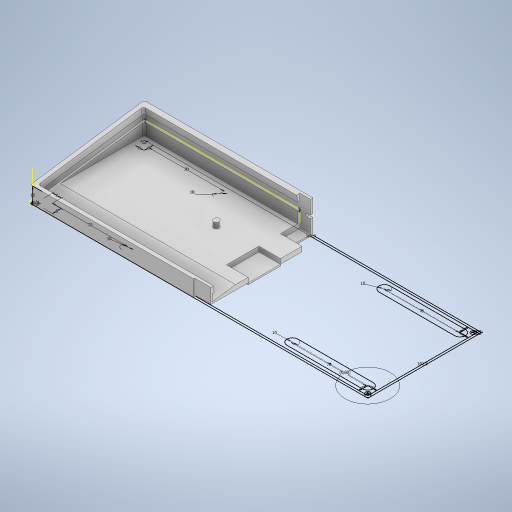
# Autodesk Inventor part: case_in_one_p1
Saved by Autodesk Inventor 2024 (Build 280153000, 153)
## iProperties
Created: 2023-08-03
Part Number: case_in_one_p1
Material: Generic
Document SubType Name: Modeling
Designer: Mika
Density: 1 g/cm^3
Appearance: Default
Author: Mika
Autodesk Inventor part; units mm, degrees
ref_plane "YZ Plane" through (0, 0, 0) normal (1, 0, 0) x (0, 1, 0)
ref_plane "XZ Plane" through (0, 0, 0) normal (0, 1, 0) x (-1, 0, 0)
ref_plane "XY Plane" through (0, 0, 0) normal (0, 0, 1) x (1, 0, 0)
sketch "Sketch1" plane through (0, 0, 0) normal (0, 1, 0) x (-1, 0, 0)
  line L0 (0, 0) -> (-2, 0)
  line L1 (-2, 0) -> (-2, -2)
  line L2 (-2, -2) -> (0, -2)
  line L3 (0, -2) -> (0, 0)
  line L4 (-2, -2) -> (-310.9, -2)
  line L5 (-310.9, -2) -> (-310.9, -103.5)
  line L6 (-308.9, -103.5) -> (-2, -103.5)
  line L7 (-2, -103.5) -> (-2, -2)
  line L8 (-310.9, -103.5) -> (-312.9, -103.5)
  line L9 (-312.9, -103.5) -> (-312.9, -105.5)
  line L10 (-312.9, -105.5) -> (-310.9, -105.5)
  line L11 (-310.9, -105.5) -> (-310.9, -103.5)
  line L12 (-312.9, -105.5) -> (0, -105.5)
  line L13 (0, -105.5) -> (0, 0)
  line L14 (0, 0) -> (-312.9, 0)
  line L15 (-312.9, 0) -> (-312.9, -105.5)
  line L16 (-2, -2) -> (-4, -2)
  line L17 (-4, -2) -> (-4, -4)
  line L18 (-4, -4) -> (-2, -4)
  line L19 (-2, -4) -> (-2, -2)
  line L20 (-2, -103.5) -> (-4, -103.5)
  line L21 (-4, -103.5) -> (-4, -101.5)
  line L22 (-4, -101.5) -> (-2, -101.5)
  line L23 (-2, -101.5) -> (-2, -103.5)
  line L24 (-310.9, -103.5) -> (-308.9, -103.5)
  line L25 (-308.9, -103.5) -> (-308.9, -101.5)
  line L26 (-308.9, -101.5) -> (-310.9, -101.5)
  line L27 (-310.9, -101.5) -> (-310.9, -103.5)
  line L28 (-310.9, -2) -> (-308.9, -2)
  line L29 (-308.9, -2) -> (-308.9, -4)
  line L30 (-308.9, -4) -> (-310.9, -4)
  line L31 (-310.9, -4) -> (-310.9, -2)
  circle A0 centre (-4, -101.5) radius 2
  circle A1 centre (-4, -4) radius 2
  circle A2 centre (-308.9, -4) radius 2
  circle A3 centre (-308.9, -101.5) radius 2
  circle A4 centre (-310.9, -103.5) radius 2
  circle A5 centre (-2, -103.5) radius 2
  circle A6 centre (-2, -2) radius 2
  circle A7 centre (-310.9, -2) radius 2
  line L32 (-2, -2) -> (-10, -2)
  line L33 (-10, -2) -> (-10, -10)
  line L34 (-10, -10) -> (-2, -10)
  line L35 (-2, -10) -> (-2, -2)
  line L36 (-310.9, -2) -> (-302.9, -2)
  line L37 (-302.9, -2) -> (-302.9, -10)
  line L38 (-302.9, -10) -> (-310.9, -10)
  line L39 (-310.9, -10) -> (-310.9, -2)
  line L40 (-310.9, -103.5) -> (-302.9, -103.5)
  line L41 (-302.9, -103.5) -> (-302.9, -95.5)
  line L42 (-302.9, -95.5) -> (-310.9, -95.5)
  line L43 (-310.9, -95.5) -> (-310.9, -103.5)
  line L44 (-2, -103.5) -> (-10, -103.5)
  line L45 (-10, -103.5) -> (-10, -95.5)
  line L46 (-10, -95.5) -> (-2, -95.5)
  line L47 (-2, -95.5) -> (-2, -103.5)
  line L48 (-10, -95.5) -> (-80, -95.5) construction
  line L49 (-10, -90.5) -> (-80, -90.5)
  line L50 (-80, -100.5) -> (-10, -100.5)
  arc A8 (-10, -100.5) -> (-10, -90.5) centre (-10, -95.5) ccw
  arc A9 (-80, -90.5) -> (-80, -100.5) centre (-80, -95.5) ccw
  line L51 (-302.9, -95.5) -> (-232.9, -95.5) construction
  line L52 (-302.9, -100.5) -> (-232.9, -100.5)
  line L53 (-232.9, -90.5) -> (-302.9, -90.5)
  arc A10 (-302.9, -90.5) -> (-302.9, -100.5) centre (-302.9, -95.5) ccw
  arc A11 (-232.9, -100.5) -> (-232.9, -90.5) centre (-232.9, -95.5) ccw
  line L54 (-302.9, -10) -> (-232.9, -10) construction
  line L55 (-302.9, -15) -> (-232.9, -15)
  line L56 (-232.9, -5) -> (-302.9, -5)
  arc A12 (-302.9, -5) -> (-302.9, -15) centre (-302.9, -10) ccw
  arc A13 (-232.9, -15) -> (-232.9, -5) centre (-232.9, -10) ccw
  line L57 (-302.9, -10) -> (-232.9, -10) construction
  line L58 (-10, -10) -> (-80, -10) construction
  line L59 (-10, -5) -> (-80, -5)
  line L60 (-80, -15) -> (-10, -15)
  arc A14 (-10, -15) -> (-10, -5) centre (-10, -10) ccw
  arc A15 (-80, -5) -> (-80, -15) centre (-80, -10) ccw
  point P0 (-2, -105.5)
  point P1 (0, -103.5)
  point P2 (-310.9, 0)
  point P3 (-312.9, -2)
  point P4 (-45, -95.5)
  point P5 (-267.9, -95.5)
  point P6 (-267.9, -10)
  point P7 (-45, -10)
  dimension "d0" = 2
  dimension "d1" = 2
  dimension "d2" = 308.9
  dimension "d3" = 101.5
  dimension "d4" = 2
  dimension "d5" = 2
  dimension "d6" = 2
  dimension "d7" = 2
  dimension "d8" = 2
  dimension "d9" = 2
  dimension "d10" = 2
  dimension "d11" = 2
  dimension "d12" = 2
  dimension "d13" = 2
  dimension "d66" = 8
  dimension "d67" = 8
  dimension "d68" = 8
  dimension "d69" = 8
  dimension "d70" = 8
  dimension "d71" = 8
  dimension "d72" = 8
  dimension "d73" = 8
  dimension "d74" = 70
  dimension "d75" = 10
  dimension "d76" = 70
  dimension "d77" = 10
  dimension "d78" = 70
  dimension "d79" = 0
  dimension "d80" = 10
  dimension "d81" = 70
  dimension "d82" = 10
  constraints: 130 end point, 29 parallel, 18 tangent, 16 point on circle, 14 horizontal, 12 perpendicular, 10 centre point, 8 coincident, 4 midpoint, 2 point on line, 1 collinear, 18 other
  measures "d0" distance of L2.end L1.end
  measures "d1" distance of L1.end L0.end
  measures "d2" distance of L6.end L5.end
  measures "d3" distance of L5.end L4.end
  measures "d4" distance of L10.end L9.end
  measures "d5" distance of L9.end L8.end
  measures "d6" distance of L18.end L17.end
  measures "d7" distance of L17.end L16.end
  measures "d8" distance of L21.end L22.end
  measures "d9" distance of L20.end L21.end
  measures "d10" distance of L26.end L25.end
  measures "d11" distance of L6.start L25.end
  measures "d12" distance of L29.end L30.end
  measures "d13" distance of L28.end L29.end
  measures "d66" distance of L34.end L33.end
  measures "d67" distance of L33.end L32.end
  measures "d68" distance of L37.end L38.end
  measures "d69" distance of L36.end L37.end
  measures "d70" distance of L42.end L41.end
  measures "d71" distance of L41.end L40.end
  measures "d72" distance of L45.end L46.end
  measures "d73" distance of L44.end L45.end
  measures "d74" distance of L45.end L48.end
  measures "d75" diameter of A9
  measures "d76" distance of L41.end L51.end
  measures "d77" diameter of A11
  measures "d78" distance of L37.end L54.end
  measures "d79" distance between parallel lines of L54 L57
  measures "d80" diameter of A13
  measures "d81" distance of L33.end L58.end
  measures "d82" diameter of A15
extrude "Extrusion1" add sketch "Sketch1" along normal blind 6 contours A1 L7 L34 A14 L33 L4 | A6 L18 L17 | L17 L18 A1 | A1 A6 | A2 L30 L29 | L4 L37 A12 L38 L5 A2 | A7 A2 | L29 L30 A7 | L33 L59 A15 L60 A14 L34 L7 L46 A8 L49 A9 L50 L45 L6 L41 L52 A11 L53 A10 L42 L5 L38 A12 L55 A13 L56 L37 L4 | A0 L6 L45 A8 L46 L7 | A5 L21 L22 | L22 L21 A0 | A0 A5 | A14 L34 L33 | L33 L34 A14 L60 A15 L59 | L56 A13 L55 A12 L38 L37 | L37 L38 A12 | A3 L25 L26 | L5 L42 A10 L41 L6 A3 | A4 A3 | L26 L25 A4 | A8 L45 L46 | L46 L45 L50 A9 L49 A8 | A10 L53 A11 L52 L41 L42 | L42 L41 A10
sketch "Sketch2" plane through (0, 6, 0) normal (0, 1, 0) x (1, 0, 0)
  arc A0 (2, 4) -> (4, 2) centre (4, 4) ccw projected
  line L0 (2, 2) -> (4, 2)
  line L1 (4, 2) -> (4, 4)
  line L2 (4, 4) -> (2, 4)
  line L3 (2, 4) -> (2, 2)
  arc A1 (310.9, 101.5) -> (308.9, 103.5) centre (308.9, 101.5) ccw projected
  line L4 (308.9, 101.5) -> (310.9, 101.5)
  line L5 (310.9, 101.5) -> (310.9, 103.5)
  line L6 (310.9, 103.5) -> (308.9, 103.5)
  line L7 (308.9, 103.5) -> (308.9, 101.5)
  line L8 (308.9, 101.5) -> (4, 101.5)
  line L9 (4, 101.5) -> (4, 4)
  line L10 (4, 4) -> (308.9, 4)
  line L11 (308.9, 4) -> (308.9, 101.5)
  line L12 (4, 101.5) -> (6, 101.5)
  line L13 (6, 101.5) -> (6, 99.5)
  line L14 (6, 99.5) -> (4, 99.5)
  line L15 (4, 99.5) -> (4, 101.5)
  line L16 (4, 4) -> (6, 4)
  line L17 (6, 4) -> (6, 6)
  line L18 (6, 6) -> (4, 6)
  line L19 (4, 6) -> (4, 4)
  line L20 (308.9, 4) -> (306.9, 4)
  line L21 (306.9, 4) -> (306.9, 6)
  line L22 (306.9, 6) -> (308.9, 6)
  line L23 (308.9, 6) -> (308.9, 4)
  line L24 (308.9, 101.5) -> (306.9, 101.5)
  line L25 (306.9, 101.5) -> (306.9, 99.5)
  line L26 (306.9, 99.5) -> (308.9, 99.5)
  line L27 (308.9, 99.5) -> (308.9, 101.5)
  circle A2 centre (306.9, 99.5) radius 2
  circle A3 centre (306.9, 6) radius 2
  circle A4 centre (6, 6) radius 2
  circle A5 centre (6, 99.5) radius 2
  line L28 (2, 2) -> (310.9, 2)
  line L29 (310.9, 2) -> (310.9, 103.5)
  line L30 (310.9, 103.5) -> (2, 103.5)
  line L31 (2, 103.5) -> (2, 2)
  line L32 (4, 101.5) -> (111, 101.5)
  line L33 (111, 101.5) -> (111, 61.5)
  line L34 (111, 61.5) -> (4, 61.5)
  line L35 (4, 61.5) -> (4, 101.5)
  line L36 (308.9, 101.5) -> (201.9, 101.5)
  line L37 (201.9, 101.5) -> (201.9, 61.5)
  line L38 (201.9, 61.5) -> (308.9, 61.5)
  line L39 (308.9, 61.5) -> (308.9, 101.5)
  circle A6 centre (111, 61.5) radius 2.5
  circle A7 centre (201.9, 61.5) radius 2.5
  point P0 (0, 0)
  dimension "d18" = 2
  dimension "d19" = 2
  dimension "d20" = 2
  dimension "d21" = 2
  dimension "d22" = 2
  dimension "d23" = 2
  dimension "d24" = 2
  dimension "d25" = 2
  dimension "d60" = 107
  dimension "d61" = 40
  dimension "d62" = 107
  dimension "d63" = 40
  dimension "d64" = 5
  dimension "d65" = 5
  constraints: 80 end point, 20 parallel, 10 horizontal, 10 perpendicular, 6 coincident, 2 centre point, 12 other
  measures "d18" distance of L13.end L14.end
  measures "d19" distance of L12.end L13.end
  measures "d20" distance of L18.end L17.end
  measures "d21" distance of L17.end L16.end
  measures "d22" distance of L21.end L22.end
  measures "d23" distance of L20.end L21.end
  measures "d24" distance of L26.end L25.end
  measures "d25" distance of L25.end L24.end
  measures "d60" distance of L33.end L34.end
  measures "d61" distance of L32.end L33.end
  measures "d62" distance of L38.end L37.end
  measures "d63" distance of L37.end L36.end
  measures "d64" diameter of A6
  measures "d65" diameter of A7
extrude "Extrusion3" add sketch "Sketch2" along normal blind 11 contours L2 L1 A0 | L31 L30 L7 L8 L9 L2 | L1 L10 L11 L4 L29 L28 | L9 A4 L10 | A1 L4 L7 | A3 L11 L10 | L11 A2 L8 | L9 L8 A5 | A6 L33 L34 | L34 L33 A6 | A7 L37 L38 | L38 L37 A7
sketch "Sketch6" plane through (4, 0, -2) normal (0, 0, 1) x (1, 0, 0)
  line L0 (0, 0) -> (0, 3)
  line L1 (0, 0) -> (0, 17) projected
  line L2 (0, 3) -> (4.2844, 3)
  point P0 (-4, 0)
  dimension "d30" = 3
  constraints: 4 end point, 1 horizontal, 1 point on line
  measures "d30" distance of L0.start L0.end
ref_plane "Work Plane3" through (4, 3, -2) normal (0, 0.9906211, 0.1366374) x (1, 0, 0)
sketch "Sketch7" plane through (4, 3, -2) normal (0, 0.9906211, 0.1366374) x (1, 0, 0)
  line L0 (-11.9738, -4.1183) -> (314.319, -4.1183)
  line L1 (314.319, -4.1183) -> (314.319, 105.2243)
  line L2 (314.319, 105.2243) -> (-11.9738, 105.2243)
  line L3 (-11.9738, 105.2243) -> (-11.9738, -4.1183)
  point P0 (-4, -2.3912)
  constraints: 8 end point, 2 parallel, 1 horizontal, 1 perpendicular
extrude "Extrusion4" cut sketch "Sketch7" along normal blind 15
extrude "Extrusion5" add sketch "Sketch1" along normal blind 30 contours A6 L2 L1 | A6 L4 A7 L14 | L1 L4 A6 | A6 L7 L2 | L13 A5 L7 A6 | L7 A1 L4 | A7 L4 L5 | A5 L6 L7 | A2 L5 L4 | A7 L5 A4 L15 | L7 L6 A0 | L12 A4 L6 A5 | A4 L5 L8 | L8 L11 A4 | L11 L24 A4 | L5 A3 L24
sketch "Sketch8" plane through (2, 0, 0) normal (0, 0, 1) x (1, 0, 0)
  line L0 (0, 0) -> (308.9, 0) projected
  line L1 (0, 0) -> (0, 15)
  line L2 (0, 0) -> (0, 30) projected
  line L3 (0, 15) -> (8.6309, 15)
  point P0 (-2, 0)
  dimension "d35" = 15
  constraints: 4 end point, 1 midpoint, 1 perpendicular
  measures "d35" distance of L0.start L1.end
ref_plane "Work Plane5" through (4, 9.439, -1.1119) normal (0, 0.9906211, 0.1366374) x (1, 0, 0)
ref_plane "Work Plane4" through (2, 15, 0) normal (0, 0.9900431, 0.1407644) x (1, 0, 0)
sketch "Sketch9" plane through (2, 15, 0) normal (0, 0.9900431, 0.1407644) x (1, 0, 0)
  line L0 (-10.8659, -4.1932) -> (315.4138, -4.1932)
  line L1 (315.4138, -4.1932) -> (315.4138, 110.562)
  line L2 (315.4138, 110.562) -> (-10.8659, 110.562)
  line L3 (-10.8659, 110.562) -> (-10.8659, -4.1932)
  point P0 (-2, -2.1115)
  constraints: 8 end point, 2 parallel, 1 horizontal, 1 perpendicular
extrude "Extrusion6" cut sketch "Sketch9" along normal blind 25
sketch "Sketch10" plane through (4, 3, -2) normal (0, 0.9906211, 0.1366374) x (1, 0, 0)
  line L0 (306.9, 100.442) -> (306.9, 2.0189) projected
  line L1 (-2, 100.442) -> (-2, 102.1783) projected
  line L2 (306.9, 100.442) -> (-2, 100.442)
  line L3 (152.45, 100.442) -> (152.45, 102.461)
  line L4 (304.9, 102.461) -> (0, 102.461) projected
  line L5 (306.9, 105.9964) -> (-2, 105.9964) projected
  line L6 (147.95, 94.8877) -> (156.95, 94.8877)
  line L7 (156.95, 94.8877) -> (156.95, 105.9964)
  line L8 (156.95, 105.9964) -> (147.95, 105.9964)
  line L9 (147.95, 105.9964) -> (147.95, 94.8877)
  line L10 (147.95, 94.8877) -> (156.95, 105.9964) construction
  line L11 (156.95, 94.8877) -> (147.95, 105.9964) construction
  line L12 (306.9, 100.442) -> (306.9, 99.411)
  line L13 (302.9, 100.442) -> (2, 100.442) projected
  line L14 (218.9, 100.442) -> (218.9, 102.2173)
  line L15 (198.9, 98.442) -> (238.9, 98.442)
  line L16 (238.9, 98.442) -> (238.9, 102.442)
  line L17 (238.9, 102.442) -> (198.9, 102.442)
  line L18 (198.9, 102.442) -> (198.9, 98.442)
  line L19 (198.9, 98.442) -> (238.9, 102.442) construction
  line L20 (238.9, 98.442) -> (198.9, 102.442) construction
  point P0 (-4, -2.3912)
  dimension "d39" = 9
  dimension "d44" = 88
  dimension "d45" = 40
  dimension "d46" = 4
  constraints: 32 end point, 6 midpoint, 4 parallel, 4 perpendicular, 3 point on line, 2 horizontal
  measures "d39" distance of L8.end L7.end
  measures "d44" distance between parallel lines of L12 L14
  measures "d45" distance of L17.end L16.end
  measures "d46" distance of L16.end L15.end
extrude "Extrusion7" cut sketch "Sketch10" against normal blind 3
sketch "Sketch12" plane through (4, 3, -2) normal (0, -0.9906211, -0.1366374) x (1, 0, 0)
  point P0 (-4, 2.3912)
extrude "Extrusion10" cut sketch "Sketch1" along normal blind 1 contours A14 L34 L33 | L33 L34 A14 L60 A15 L59 | L56 A13 L55 A12 L38 L37 | L37 L38 A12 | A8 L45 L46 | L46 L45 L50 A9 L49 A8 | A10 L53 A11 L52 L41 L42 | L42 L41 A10
fillet "Fillet2" radius 1 6 edges at (151.95, 13.9696, -103.5) (160.95, 13.9696, -103.5) (160.95, 17.1399, -104.5) (160.95, 17, -103.5) (151.95, 17.1399, -104.5) (151.95, 17, -103.5)
sketch "Sketch15" plane through (0, 0, 0) normal (0, -1, 0) x (1, 0, 0)
  line L0 (152.95, -105.5) -> (159.95, -105.5) projected
  line L1 (156.45, -105.5) -> (156.45, -85.5)
  line L2 (156.45, -85.5) -> (146.45, -85.5)
  line L3 (146.45, -85.5) -> (146.45, -65.5)
  line L4 (146.45, -65.5) -> (166.45, -65.5)
  line L5 (166.45, -65.5) -> (166.45, -35.5)
  line L6 (166.45, -35.5) -> (151.45, -35.5)
  line L7 (151.45, -35.5) -> (151.45, 0)
  line L8 (308.9, -2) -> (4, -2) projected
  line L9 (0, -105.5) -> (0, 0)
  line L10 (0, 0) -> (312.8991, 0)
  line L11 (312.8991, 0) -> (312.8991, -105.5)
  line L12 (156.45, -105.5) -> (156.45, -103.5)
  line L13 (308.9, -103.5) -> (4, -103.5) projected
  line L14 (156.45, -105.5) -> (156.45, -107.5)
  line L15 (151.45, 0) -> (151.45, 2)
  line L16 (314.6953, -107.5) -> (-5.5477, -107.5)
  line L17 (-5.5477, -107.5) -> (-5.5477, 1.9279)
  line L18 (-5.5477, 1.9279) -> (314.6953, 1.9279)
  line L19 (314.6953, 1.9279) -> (314.6953, -107.5)
  point P0 (151.45, 1.9279)
  dimension "d86" = 20
  dimension "d87" = 10
  dimension "d88" = 20
  dimension "d89" = 20
  dimension "d90" = 30
  dimension "d91" = 15
  dimension "d92" = 2
  dimension "d93" = 2
  dimension "d94" = 2
  constraints: 34 end point, 7 perpendicular, 3 parallel, 3 vertical, 2 midpoint, 1 horizontal
  measures "d86" distance of L1.start L1.end
  measures "d87" distance of L1.end L2.end
  measures "d88" distance of L2.end L3.end
  measures "d89" distance of L3.end L4.end
  measures "d90" distance of L4.end L5.end
  measures "d91" distance of L5.end L6.end
  measures "d92" distance of L1.start L12.end
  measures "d93" distance of L1.start L14.end
  measures "d94" distance of L7.end L15.end
extrude "Extrusion11" cut sketch "Sketch15" against normal blind 30.75 contours L1 L2 L3 L4 L5 L6 L7 L15 L18 L19 L16 L14
sketch "Sketch16" plane through (166.45, 0, -35.5) normal (1, 0, 0) x (0, 0, -1)
  line L0 (-35.5, 1.5) -> (-33.5, 1.5) projected
  line L1 (-33.5, 1.5) -> (68, 1.5) projected
  line L2 (-34.5, 1.5) -> (68, 1.5)
  line L3 (-34.5, 1.5) -> (-34.5, 18.0111)
  line L4 (68, 1.5) -> (68, 37.3822)
  line L5 (68, 0) -> (68, 29.7156) projected
  line L6 (68, 37.3822) -> (66, 37.3822)
  line L7 (66, 6) -> (64, 6) projected
  line L8 (66, 37.3822) -> (66, 6)
  line L9 (66, 6) -> (-31.5124, 6)
  line L10 (-31.5124, 6) -> (-31.5124, 18.0111)
  line L11 (-31.5124, 18.0111) -> (-34.5, 18.0111)
  line L12 (0, 0) -> (0, 6) projected
  line L13 (0, 6) -> (0, 3)
  line L14 (30, 0) -> (30, 6) projected
  line L15 (30, 6) -> (30, 3)
  line L16 (50, 6) -> (66, 6) projected
  line L17 (50, 6) -> (50, 1.5)
  point P0 (-35.5, 0)
  point P1 (68, 28.2006)
  point P2 (30, 1.5)
  point P3 (0, 1.5)
  constraints: 22 end point, 6 perpendicular, 3 midpoint, 2 collinear, 1 point on line, 1 vertical
extrude "Extrusion12" cut sketch "Sketch16" against normal blind 20 contours L12 L9 L14 L1 | L17 L9 L7 L8 L6 L4 L1
extrude "Extrusion13" add sketch "Sketch16" against normal blind 20 contours L14 L9 L17 L1
sketch "Sketch18" plane through (4, 17, -103.5) normal (0, 0, 1) x (1, 0, 0)
  line L0 (142.45, 0) -> (0, 0) projected
  line L1 (0, 0) -> (0, -2)
  line L2 (0, -11) -> (0, -0.5517) projected
  line L3 (142.45, 0) -> (142.45, -2)
  line L4 (142.45, -11) -> (142.45, -0.2759) projected
  point P0 (-4, -17)
  dimension "d104" = 2
  dimension "d105" = 2
  constraints: 4 end point, 2 point on line
  measures "d104" distance of L0.end L1.end
  measures "d105" distance of L0.start L3.end
sketch "Sketch20" plane through (4, 9.439, -1.1119) normal (0, 0.9906211, 0.1366374) x (1, 0, 0)
  line L0 (2, 101.3417) -> (142.45, 101.3417)
  line L1 (142.45, 102.461) -> (0, 102.461) projected
  line L2 (142.45, 101.3417) -> (142.45, 104.2831)
  line L3 (142.45, 104.2831) -> (-2.4512, 104.2831)
  line L4 (-2.4512, 104.2831) -> (-2.4512, 0.4321)
  line L5 (-4, 1.6785) -> (-4, 104.1984) projected
  line L6 (-2.4512, 0.4321) -> (147.45, 0.4321)
  line L7 (147.45, -0.3416) -> (147.45, 1.6785) projected
  line L8 (147.45, 0.4321) -> (147.45, 0.894)
  line L9 (147.45, 0.894) -> (147.45, 2.894)
  line L10 (147.45, 2.894) -> (0.0009, 2.894)
  line L11 (0.0009, 2.894) -> (0.0009, 101.3417)
  line L12 (0.0009, 101.3417) -> (2, 101.3417)
  point P0 (-4, -2.3912)
  dimension "d110" = 2
  constraints: 20 end point, 5 perpendicular, 4 point on line, 3 parallel
  measures "d110" distance of L8.end L9.end
extrude "Extrusion16" add sketch "Sketch20" along normal blind 6.1
fillet "Fillet3" radius 2 2 edges at (4.0009, 26.3075, -101.0863) (4.0009, 12.8559, -3.5619)
sketch "Sketch21" plane through (2, 15, 0) normal (0, 0.9900431, 0.1407644) x (1, 0, 0)
  line L0 (-11.1618, 110.2013) -> (188.4108, 110.2013)
  line L1 (188.4108, 110.2013) -> (188.4108, -4.9713)
  line L2 (188.4108, -4.9713) -> (-11.1618, -4.9713)
  line L3 (-11.1618, -4.9713) -> (-11.1618, 110.2013)
  point P0 (-2, -2.1115)
  constraints: 8 end point, 2 parallel, 1 horizontal, 1 perpendicular
extrude "Extrusion17" cut sketch "Sketch21" along normal blind 6.1
sketch "Sketch22" plane through (151.45, 0, 0) normal (1, 0, 0) x (0, 0, -1)
  line L0 (0, 0) -> (0, 15) projected
  line L1 (3.2034, 15.4555) -> (3.9787, 9.8345) projected
  line L2 (0, 15) -> (3.2034, 15.4555)
  line L3 (3.2034, 15.4555) -> (3.9787, 9.8345)
  line L4 (3.9787, 9.8345) -> (2, 9.5615)
  line L5 (2, 0) -> (2, 15.2844) projected
  line L6 (0, 15) -> (0, 0)
  line L7 (2, 0) -> (0, 0) projected
  line L8 (35.5, 0) -> (35.5, 1.5) projected
  line L9 (0, 0) -> (35.5, 0)
  line L10 (35.5, 0) -> (35.5, 7.6207)
  line L11 (99.5, 16.4483) -> (23.75, 6) projected
  line L12 (35.5, 7.6207) -> (2, 3)
  line L13 (2, 3) -> (2, 9.5615)
  line L14 (23.75, 6) -> (35.5, 6)
  line L15 (99.5, 6) -> (23.75, 6) projected
  line L16 (35.5, 1.5) -> (1, 1.5)
  line L17 (1, 1.5) -> (1, 15.1422)
  dimension "d118" = 1
  constraints: 22 end point, 5 point on line, 4 perpendicular, 2 collinear, 1 horizontal, 1 parallel, 1 vertical
  measures "d118" distance between parallel lines of L0 L17
extrude "Extrusion18" add sketch "Sketch22" along normal blind 15 contours L2 L5 L16 L17 | L5 L12 L14 L10 L16 | L2 L1 L4 L5
body "Solid1"
